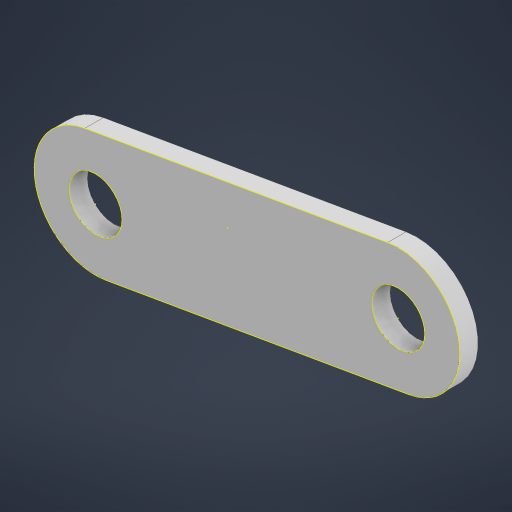
# Autodesk Inventor part: shaft-retainer
Saved by Autodesk Inventor 2024 (Build 280153000, 153)
## iProperties
Created: 2023-04-20
Part Number: shaft-retainer
Material: Generic
Document SubType Name: Modeling
Designer: liamt
Density: 1 g/cm^3
Appearance: Default
Author: liamt
Autodesk Inventor part; units mm, degrees
ref_plane "YZ Plane" through (0, 0, 0) normal (1, 0, 0) x (0, 1, 0)
ref_plane "XZ Plane" through (0, 0, 0) normal (0, 1, 0) x (-1, 0, 0)
ref_plane "XY Plane" through (0, 0, 0) normal (0, 0, 1) x (1, 0, 0)
sketch "Sketch1" plane through (0, 0, 0) normal (0, 0, 1) x (1, 0, 0)
  circle A0 centre (-10.9262, -3.7547) radius 2.1844
  circle A1 centre (14.1012, 0.5797) radius 2.1844
  line L0 (-11.7931, 1.2507) -> (13.2343, 5.5852)
  line L1 (-10.0593, -8.7602) -> (14.9681, -4.4257)
  arc A2 (-11.7931, 1.2507) -> (-10.0593, -8.7602) centre (-10.9262, -3.7547) ccw
  arc A3 (14.9681, -4.4257) -> (13.2343, 5.5852) centre (14.1012, 0.5797) ccw
  point P0 (0, 0)
  dimension "d7" = 25.4
  constraints: 4 centre point, 4 end point, 4 point on circle, 4 tangent, 5 other
  measures "d7" distance of L0.start L0.end
extrude "Extrusion1" add sketch "Sketch1" along normal blind 1.524
sketch "Sketch2" plane through (0, 0, 1.524) normal (0, 0, 1) x (1, 0, 0)
  arc A0 (14.9681, -4.4257) -> (13.2343, 5.5852) centre (14.1012, 0.5797) ccw projected
  line L0 (13.2343, 5.5852) -> (-11.7931, 1.2507) projected
  arc A1 (-11.7931, 1.2507) -> (-10.0593, -8.7602) centre (-10.9262, -3.7547) ccw projected
  line L1 (-10.0593, -8.7602) -> (14.9681, -4.4257) projected
  circle A2 centre (14.1012, 0.5797) radius 2.1844 projected
  circle A3 centre (-10.9262, -3.7547) radius 2.1844 projected
  point P0 (0, 0)
body "Solid1"
